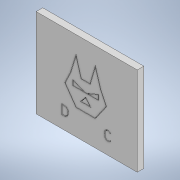
# Autodesk Inventor part: Tablero_DC_007
Saved by Autodesk Inventor 2022 (Build 260153000, 153)
## iProperties
Created: 2022-09-01
Part Number: Tablero_DC_007
Material: Generic
Document SubType Name: Modeling
Designer: Asus
Density: 1 g/cm^3
Appearance: Default
Author: Asus
Autodesk Inventor part; units mm, degrees
ref_plane "YZ Plane" through (0, 0, 0) normal (1, 0, 0) x (0, 1, 0)
ref_plane "XZ Plane" through (0, 0, 0) normal (0, 1, 0) x (-1, 0, 0)
ref_plane "XY Plane" through (0, 0, 0) normal (0, 0, 1) x (1, 0, 0)
sketch "Sketch1" plane through (0, 0, 0) normal (0, 0, 1) x (1, 0, 0)
  line L0 (0, 0) -> (308, 0)
  line L1 (308, 0) -> (308, 270)
  line L2 (308, 270) -> (0, 270)
  line L3 (0, 270) -> (0, 0)
  dimension "d0" = 308
  dimension "d1" = 270
  constraints: 8 end point, 2 parallel, 1 horizontal, 1 perpendicular
  measures "d0" distance of L2.end L1.end
  measures "d1" distance of L1.end L0.end
extrude "Extrusion1" add sketch "Sketch1" along normal blind 20
sketch "Sketch2" plane through (0, 0, 20) normal (0, 0, 1) x (1, 0, 0)
  line L0 (150.8623, 77.3843) -> (180.284, 77.3843)
  line L1 (180.284, 77.3843) -> (214.6934, 126.131)
  line L2 (214.6934, 126.131) -> (197.4887, 161.9741)
  line L3 (197.4887, 161.9741) -> (180.284, 217.8894)
  line L4 (180.284, 217.8894) -> (163.9156, 161.9741)
  line L5 (163.9156, 161.9741) -> (150.8623, 161.9741)
  line L6 (150.8623, 161.9741) -> (150.8623, 77.3843) construction
  line L7 (150.8623, 77.3843) -> (121.4405, 77.3843)
  line L8 (121.4405, 77.3843) -> (87.0311, 126.131)
  line L9 (87.0311, 126.131) -> (104.2358, 161.9741)
  line L10 (104.2358, 161.9741) -> (121.4405, 217.8894)
  line L11 (121.4405, 217.8894) -> (137.8089, 161.9741)
  line L12 (137.8089, 161.9741) -> (150.8623, 161.9741)
  line L13 (308, 0) -> (308, 270) projected
  line L14 (144.5227, 131.6434) -> (112.8382, 144.3477)
  line L15 (112.8382, 144.3477) -> (112.8382, 131.6434)
  line L16 (112.8382, 131.6434) -> (144.5227, 131.6434)
  line L17 (157.2018, 131.6434) -> (188.8863, 144.3477)
  line L18 (188.8863, 144.3477) -> (188.8863, 131.6434)
  line L19 (188.8863, 131.6434) -> (157.2018, 131.6434)
  line L20 (150.8623, 117.5428) -> (137.8089, 101.7577)
  line L21 (137.8089, 101.7577) -> (163.9156, 101.7577)
  line L22 (163.9156, 101.7577) -> (150.8623, 117.5428)
  line L23 (212.9598, 126.2762) -> (179.5067, 78.8843)
  line L24 (179.5067, 78.8843) -> (150.8623, 78.8843)
  line L25 (150.8623, 78.8843) -> (122.2178, 78.8843)
  line L26 (122.2178, 78.8843) -> (88.7647, 126.2762)
  line L27 (88.7647, 126.2762) -> (105.6366, 161.426)
  line L28 (105.6366, 161.426) -> (121.4047, 212.6725)
  line L29 (121.4047, 212.6725) -> (136.6851, 160.4741)
  line L30 (136.6851, 160.4741) -> (150.8623, 160.4741)
  line L31 (150.8623, 160.4741) -> (165.0395, 160.4741)
  line L32 (165.0395, 160.4741) -> (180.3198, 212.6725)
  line L33 (180.3198, 212.6725) -> (196.0879, 161.426)
  line L34 (196.0879, 161.426) -> (212.9598, 126.2762)
  line L35 (111.3382, 146.5653) -> (150.8623, 130.7176)
  line L36 (152.2942, 130.1434) -> (111.3382, 130.1434)
  line L37 (111.3382, 130.1434) -> (111.3382, 146.5653)
  line L38 (150.8623, 130.7176) -> (190.3863, 146.5653)
  line L39 (190.3863, 146.5653) -> (190.3863, 130.1434)
  line L40 (190.3863, 130.1434) -> (149.4303, 130.1434)
  line L41 (150.8623, 119.8965) -> (134.6221, 100.2577)
  line L42 (134.6221, 100.2577) -> (167.1025, 100.2577)
  line L43 (167.1025, 100.2577) -> (150.8623, 119.8965)
  line L44 (74.5244, 66.3096) -> (229.3713, 66.3096) construction
  line L45 (229.3713, 66.3096) -> (229.3713, 36.329) construction
  line L46 (229.3713, 36.329) -> (74.5244, 36.329) construction
  line L47 (74.5244, 36.329) -> (74.5244, 66.3096) construction
  line L48 (208.446, 49.8524) -> (208.446, 52.8954)
  line L49 (97.2006, 52.8954) -> (97.2006, 49.8524)
  spline S0 degree 2 poles (98.2109, 52.4396) (98.2109, 45.1875) (95.3431, 41.5752) knots 0 0 0 1 1 1
  spline S1 degree 2 poles (95.3431, 41.5752) (92.9717, 38.5145) (88.0359, 37.5494) knots 0 0 0 1 1 1
  spline S2 degree 2 poles (88.0359, 37.5494) (85.0303, 36.9703) (78.0264, 36.9703) knots 0 0 0 1 1 1
  line L50 (78.0264, 36.9703) -> (78.0264, 66.3096)
  spline S3 degree 2 poles (78.0264, 66.3096) (88.4219, 66.3096) (92.1169, 64.5724) knots 0 0 0 1 1 1
  spline S4 degree 2 poles (92.1169, 64.5724) (98.2109, 61.7598) (98.2109, 52.4396) knots 0 0 0 1 1 1
  spline S5 degree 2 poles (96.0877, 52.4396) (96.0877, 60.2707) (91.0139, 62.78) knots 0 0 0 1 1 1
  spline S6 degree 2 poles (91.0139, 62.78) (88.0359, 64.1863) (80.1496, 64.1863) knots 0 0 0 1 1 1
  line L51 (80.1496, 64.1863) -> (80.1496, 39.0935)
  spline S7 degree 2 poles (80.1496, 39.0935) (87.9808, 39.0935) (91.0139, 40.7756) knots 0 0 0 1 1 1
  spline S8 degree 2 poles (91.0139, 40.7756) (96.0877, 43.5882) (96.0877, 52.4396) knots 0 0 0 1 1 1
  spline S9 degree 2 poles (227.425, 41.0513) (225.219, 38.4042) (221.0277, 36.3912) (218.1599, 36.3912) knots 0 0 0 1 2 2 2
  spline S10 degree 2 poles (218.1599, 36.3912) (213.4998, 36.3912) (207.5713, 44.7463) (207.5713, 51.6951) knots 0 0 0 1 2 2 2
  spline S11 degree 2 poles (207.5713, 51.6951) (207.5713, 59.2781) (211.1284, 63.1385) knots 0 0 0 1 1 1
  spline S12 degree 2 poles (211.1284, 63.1385) (214.0238, 66.3096) (218.1599, 66.3096) knots 0 0 0 1 1 1
  spline S13 degree 2 poles (218.1599, 66.3096) (221.331, 66.3096) (225.219, 64.1863) (226.6804, 61.5392) knots 0 0 0 1 2 2 2
  spline S14 degree 2 poles (226.6804, 61.5392) (226.8459, 61.291) (226.8459, 61.0153) knots 0 0 0 1 1 1
  spline S15 degree 2 poles (226.8459, 61.0153) (226.8459, 59.9674) (225.7429, 59.9674) knots 0 0 0 1 1 1
  spline S16 degree 2 poles (225.7429, 59.9674) (225.219, 59.9674) (224.8881, 60.4913) knots 0 0 0 1 1 1
  spline S17 degree 2 poles (224.8881, 60.4913) (222.7649, 64.1863) (218.2702, 64.1863) knots 0 0 0 1 1 1
  spline S18 degree 2 poles (218.2702, 64.1863) (214.8786, 64.1863) (212.5623, 61.4289) knots 0 0 0 1 1 1
  spline S19 degree 2 poles (212.5623, 61.4289) (209.6946, 58.0372) (209.6946, 51.6951) knots 0 0 0 1 1 1
  spline S20 degree 2 poles (209.6946, 51.6951) (209.6946, 45.932) (214.6855, 38.5145) (218.2702, 38.5145) knots 0 0 0 1 2 2 2
  spline S21 degree 2 poles (218.2702, 38.5145) (222.6821, 38.5145) (225.7429, 42.43) knots 0 0 0 1 1 1
  spline S22 degree 2 poles (225.7429, 42.43) (226.0462, 42.8437) (226.5977, 42.8437) knots 0 0 0 1 1 1
  spline S23 degree 2 poles (226.5977, 42.8437) (227.7007, 42.8437) (227.7007, 41.7407) knots 0 0 0 1 1 1
  spline S24 degree 2 poles (227.7007, 41.7407) (227.7007, 41.3546) (227.425, 41.0513) knots 0 0 0 1 1 1
  point P0 (0, 0)
  point P1 (150.8623, 130.1434)
  dimension "d5" = 1.5
  dimension "d6" = 1.5
  dimension "d7" = 1.5
  dimension "d8" = 1.5
  constraints: 90 end point, 8 symmetric about line, 3 horizontal, 3 perpendicular, 2 point on line, 1 parallel, 1 vertical, 17 other
  measures "d5" distance between parallel lines of L1 L23
  measures "d6" distance between parallel lines of L14 L35
  measures "d7" distance between parallel lines of L19 L40
  measures "d8" distance between parallel lines of L22 L43
extrude "Extrusion2" cut sketch "Sketch2" against normal blind 8
body "Solid1"
